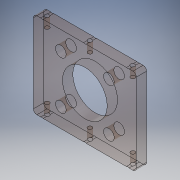
# Autodesk Inventor part: ハンド_エアシリンダ固定具
Saved by Autodesk Inventor 2019.4 (Build 234330000, 330)
## iProperties
Created: 2021-12-26
Part Number: ハンド_エアシリンダ固定具
Material: ポリカーボネート、スモーク
Document SubType Name: Modeling
Designer: 堀川皓史
Density: 1.2 g/cm^3
Appearance: ポリカーボネート - スモーク
Author: 堀川皓史
Autodesk Inventor part; units mm, degrees
ref_plane "YZ Plane" through (0, 0, 0) normal (1, 0, 0) x (0, 1, 0)
ref_plane "XZ Plane" through (0, 0, 0) normal (0, 1, 0) x (-1, 0, 0)
ref_plane "XY Plane" through (0, 0, 0) normal (0, 0, 1) x (1, 0, 0)
sketch "スケッチ1" plane through (0, 0, 0) normal (0, 0, 1) x (1, 0, 0)
  circle A0 centre (0, 0) radius 13
  circle A1 centre (-14, 14) radius 3.1
  circle A2 centre (14, 14) radius 3.1
  circle A3 centre (-14, -14) radius 3.1
  circle A4 centre (14, -14) radius 3.1
  line L0 (20, 20) -> (-20, 20) construction
  line L1 (-20, 20) -> (-20, -20) construction
  line L2 (-20, -20) -> (20, -20) construction
  line L3 (20, -20) -> (20, 20) construction
  line L4 (20, 20) -> (-20, -20) construction
  line L5 (-20, 20) -> (20, -20) construction
  line L6 (30, 25) -> (25.7483, 25)
  line L7 (-30, 25) -> (-30, -25)
  line L8 (-30, -25) -> (-25.7483, -25)
  line L9 (30, -25) -> (30, 25)
  line L10 (30, 25) -> (-30, -25) construction
  line L11 (-30, 25) -> (30, -25) construction
  arc A5 (-0.7483, 25) -> (0.7483, 25) centre (0, 26.3) ccw
  arc A6 (-25.7483, 25) -> (-24.2517, 25) centre (-25, 26.3) ccw
  arc A7 (24.2517, 25) -> (25.7483, 25) centre (25, 26.3) ccw
  arc A8 (-24.2517, -25) -> (-25.7483, -25) centre (-25, -26.3) ccw
  arc A9 (0.7483, -25) -> (-0.7483, -25) centre (0, -26.3) ccw
  arc A10 (25.7483, -25) -> (24.2517, -25) centre (25, -26.3) ccw
  arc A11 (-24.2517, 25) -> (-25.7483, 25) centre (-25, 26.3) ccw construction
  arc A12 (0.7483, 25) -> (-0.7483, 25) centre (0, 26.3) ccw construction
  arc A13 (25.7483, 25) -> (24.2517, 25) centre (25, 26.3) ccw construction
  arc A14 (-25.7483, -25) -> (-24.2517, -25) centre (-25, -26.3) ccw construction
  arc A15 (-0.7483, -25) -> (0.7483, -25) centre (0, -26.3) ccw construction
  arc A16 (24.2517, -25) -> (25.7483, -25) centre (25, -26.3) ccw construction
  line L12 (-24.2517, 25) -> (-25.7483, 25) construction
  line L13 (-25.7483, 25) -> (-30, 25)
  line L14 (-0.7483, 25) -> (-24.2517, 25)
  line L15 (0.7483, 25) -> (-0.7483, 25) construction
  line L16 (25.7483, 25) -> (24.2517, 25) construction
  line L17 (24.2517, 25) -> (0.7483, 25)
  line L18 (-24.2517, -25) -> (-0.7483, -25)
  line L19 (-25.7483, -25) -> (-24.2517, -25) construction
  line L20 (0.7483, -25) -> (24.2517, -25)
  line L21 (-0.7483, -25) -> (0.7483, -25) construction
  line L22 (25.7483, -25) -> (30, -25)
  line L23 (24.2517, -25) -> (25.7483, -25) construction
  dimension "d0" = 26
  dimension "d1" = 6.2
  dimension "d2" = 6.2
  dimension "d3" = 6.2
  dimension "d4" = 6.2
  dimension "d5" = 28
  dimension "d6" = 28
  dimension "d7" = 14
  dimension "d8" = 14
  dimension "d9" = 40
  dimension "d10" = 40
  dimension "d11" = 10
  dimension "d12" = 5
  dimension "d13" = 3
  dimension "d14" = 3
  dimension "d15" = 3
  dimension "d16" = 3
  dimension "d17" = 3
  dimension "d18" = 3
  dimension "d19" = 1.3
  dimension "d20" = 1.3
  dimension "d21" = 25
  dimension "d22" = 25
  constraints: 52 parallel, 48 end point, 24 point on circle, 17 centre point, 8 horizontal, 8 perpendicular, 8 point on line, 7 midpoint, 6 horizontal alignment, 6 vertical alignment, 2 coincident
  measures "d0" diameter of A0
  measures "d1" diameter of A1
  measures "d2" diameter of A2
  measures "d3" diameter of A3
  measures "d4" diameter of A4
  measures "d5" distance of A3.centre A1.centre
  measures "d6" distance of A1.centre A2.centre
  measures "d7" horizontal distance of point (0, 0) A1.centre
  measures "d8" horizontal distance of point (0, 0) A1.centre
  measures "d9" distance of L2.end L1.end
  measures "d10" distance of L1.end L1.start
  measures "d11" distance between parallel lines of L1 L7
  measures "d12" distance between parallel lines of L0 L6
  measures "d13" diameter of A5
  measures "d14" diameter of A6
  measures "d15" diameter of A7
  measures "d16" diameter of A8
  measures "d17" diameter of A9
  measures "d18" diameter of A10
  measures "d19" distance from line of L6 A6.centre
  measures "d20" distance from line of L8 A8.centre
  measures "d21" distance of A5.centre A6.centre
  measures "d22" distance of A5.centre A7.centre
extrude "押し出し1" add sketch "スケッチ1" along normal blind 6
sketch "スケッチ2" plane through (-24.2517, 25, 0) normal (0, 1, 0) x (1, 0, 0)
  circle A0 centre (-0.7483, -3) radius 1.25
  circle A1 centre (24.2517, -3) radius 1.25
  circle A2 centre (49.2517, -3) radius 1.25
  point P0 (24.2517, 0)
  dimension "d25" = 2.5
  dimension "d26" = 2.5
  dimension "d27" = 2.5
  dimension "d28" = 25
  dimension "d29" = 25
  dimension "d30" = 3
  constraints: 3 centre point, 2 horizontal alignment, 1 vertical alignment
  measures "d25" diameter of A0
  measures "d26" diameter of A1
  measures "d27" diameter of A2
  measures "d28" distance of A0.centre A1.centre
  measures "d29" distance of A2.centre A1.centre
  measures "d30" distance of point (24.252, 0) A1.centre
extrude "押し出し2" cut sketch "スケッチ2" against normal blind 6
sketch "スケッチ3" plane through (-24.2517, -25, 0) normal (0, -1, 0) x (1, 0, 0)
  circle A0 centre (24.2517, 3) radius 1.25 projected
  circle A1 centre (-0.7483, 3) radius 1.25 projected
  circle A2 centre (49.2517, 3) radius 1.25 projected
  point P0 (24.2517, 0)
extrude "押し出し3" cut sketch "スケッチ3" against normal blind 6
fillet "フィレット1" radius 2 4 edges at (-30, 25, 3) (30, 25, 3) (30, -25, 3) (-30, -25, 3)
equation "\"d7\" = 0.5 * d5"
equation "\"d8\" = 0.5 * d6"
